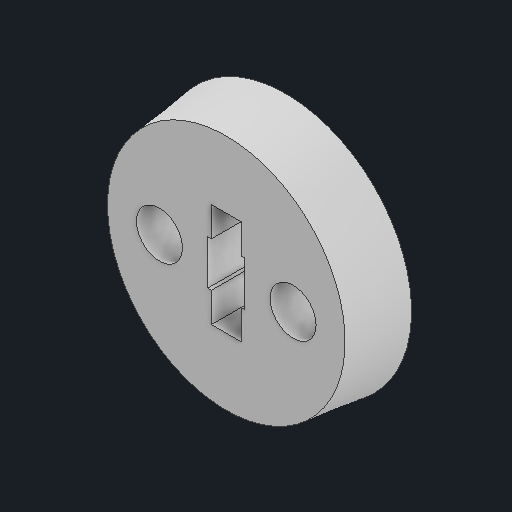
# Autodesk Inventor part: Pot_holder
Saved by Autodesk Inventor 2026.1 (Build 301233000, 233)
## iProperties
Created: 2025-11-11
Part Number: Pot_holder
Material: Generic
Document SubType Name: Modeling
Designer: Mikke
Density: 1 g/cm^3
Appearance: Default
Author: Mikke
Autodesk Inventor part; units mm, degrees
ref_plane "YZ Plane" through (0, 0, 0) normal (1, 0, 0) x (0, 1, 0)
ref_plane "XZ Plane" through (0, 0, 0) normal (0, 1, 0) x (-1, 0, 0)
ref_plane "XY Plane" through (0, 0, 0) normal (0, 0, 1) x (1, 0, 0)
sketch "Sketch1" plane through (0, 0, 0) normal (0, 0, 1) x (1, 0, 0)
  circle A0 centre (-10.6, 0) radius 8.475
  circle A1 centre (-15.1, 0) radius 2.2 projected
  circle A2 centre (-6.1, 0) radius 2.2 projected
  circle A3 centre (-10.6, 0) radius 8.475
  circle A4 centre (-15.1, 0) radius 2.2
  circle A5 centre (-6.1, 0) radius 2.2
  circle A6 centre (-15.1, 0) radius 1.55
  circle A7 centre (-6.1, 0) radius 1.55
  point P0 (0, 0)
  dimension "d9" = 3.1
  dimension "d10" = 3.1
  constraints: 6 centre point, 5 coincident, 3 concentric, 2 other
  measures "d9" diameter of A6
  measures "d10" diameter of A7
sketch "Sketch2" plane through (0, 0, 0) normal (0, 1, 0) x (-1, 0, 0)
  line L0 (19.075, 0) -> (2.125, 0) projected
  line L1 (7.55, 0) -> (13.65, 0)
  arc A0 (18.6, 4) -> (19.075, 0) centre (62.4336, 7.177) ccw
  line L2 (13.65, 0) -> (19.075, 0)
  line L3 (10.6, 0) -> (10.6, 4)
  line L4 (10.6, 0) -> (10.6, 4)
  line L5 (10.6, 4) -> (18.6, 4)
  point P0 (0, 0)
  dimension "d15" = 4
  dimension "d16" = 8
  constraints: 10 end point, 2 coincident, 2 midpoint, 2 point on circle, 2 vertical, 1 centre point, 1 collinear, 1 horizontal, 1 point on line
  measures "d15" distance of L3.start L3.end
  measures "d16" distance of L3.end L5.end
revolve "Revolution1" add sketch "Sketch2" angle 360 about axis through (-10.6, 0, 0) along (0, 0, 1)
extrude "Extrusion3" cut sketch "Sketch1" along normal blind 4 contours A6 | A7
sketch "Sketch5" plane through (-10.6, 0, 4) normal (0, 0, 1) x (1, 0, 0)
  line L0 (1, -3.5) -> (-1, -3.5)
  line L1 (-1, -3.5) -> (-1, 3.5)
  line L2 (-1, 3.5) -> (1, 3.5)
  line L3 (1, 3.5) -> (1, -3.5)
  line L4 (1, -3.5) -> (-1, 3.5) construction
  line L5 (-1, -3.5) -> (1, 3.5) construction
  circle A0 centre (-4.5, 0) radius 1.55 projected
  circle A1 centre (4.5, 0) radius 1.55 projected
  circle A2 centre (-4.5, 0) radius 3
  circle A3 centre (4.5, 0) radius 3
  line L6 (1.25, -1.5) -> (-1.25, -1.5)
  line L7 (-1.25, -1.5) -> (-1.25, 1.5)
  line L8 (-1.25, 1.5) -> (1.25, 1.5)
  line L9 (1.25, 1.5) -> (1.25, -1.5)
  line L10 (1.25, -1.5) -> (-1.25, 1.5) construction
  line L11 (-1.25, -1.5) -> (1.25, 1.5) construction
  point P0 (10.6, 0)
  point P1 (0, 0)
  point P2 (1, -1.5)
  point P3 (1, 1.5)
  point P4 (-1, 1.5)
  point P5 (-1, -1.5)
  dimension "d17" = 2
  dimension "d18" = 7
  dimension "d19" = 6
  dimension "d20" = 6
  dimension "d21" = 2.5
  dimension "d22" = 3
  constraints: 24 end point, 4 midpoint, 4 parallel, 2 centre point, 2 coincident, 2 horizontal, 2 perpendicular
  measures "d17" distance of L1.end L2.end
  measures "d18" distance of L0.end L1.end
  measures "d19" diameter of A2
  measures "d20" diameter of A3
  measures "d21" distance of L7.end L8.end
  measures "d22" distance of L6.end L7.end
extrude "Extrusion5" cut sketch "Sketch5" against normal blind 4 contours L0 L1 L6 L3 | L6 L1 L8 L3 | L3 L8 L9 L6 | L6 L7 L8 L1 | L8 L1 L2 L3
body "Solid1"
